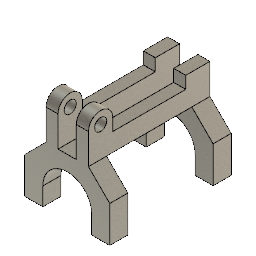
ch4Excercises v7 (Autodesk Fusion 360 design; units mm, degrees)
Autodesk Fusion 360 part; units mm, degrees
note: some values were not read from the file. Chosen so that the rebuilt part matches the saved one: which face or edge a step refers to.
sketch "Sketch1" plane through (0, 0, 0) normal (0, 0, 1) x (1, 0, 0) in component "ch4-1"
  line L0 (0, 0) -> (25.4, 0)
  line L1 (25.4, 0) -> (31.75, 6.35)
  line L2 (25.4, 0) -> (41.3581, 0) construction
  line L3 (31.75, 6.35) -> (31.75, 9.525)
  line L4 (31.75, 9.525) -> (19.05, 9.525)
  line L5 (19.05, 9.525) -> (19.05, 5.08)
  line L6 (0, 0) -> (-6.35, 6.35)
  line L7 (0, 0) -> (10.2611, 0) construction
  line L8 (-6.35, 6.35) -> (-6.35, 25.4)
  line L9 (-6.35, 25.4) -> (0, 31.75)
  line L10 (0, 31.75) -> (25.4, 31.75)
  line L11 (25.4, 31.75) -> (31.75, 25.4)
  line L12 (25.4, 31.75) -> (30.3579, 31.75) construction
  line L13 (31.75, 25.4) -> (31.75, 22.225)
  line L14 (31.75, 22.225) -> (19.05, 22.225)
  line L15 (19.05, 22.225) -> (19.05, 26.67)
  line L16 (19.05, 26.67) -> (4.445, 26.67)
  line L17 (4.445, 26.67) -> (1.27, 23.495)
  line L18 (1.27, 23.495) -> (1.27, 8.255)
  line L19 (1.27, 8.255) -> (4.445, 5.08)
  line L20 (4.445, 5.08) -> (19.05, 5.08)
  dimension "d17" = 25.4
  dimension "d18" = 45
  dimension "d20" = 6.35
  dimension "d21" = 9.525
  dimension "d22" = 12.7
  dimension "d23" = 5.08
  dimension "d24" = 135
  dimension "d26" = 6.35
  dimension "d27" = 6.35
  dimension "d28" = 31.75
  dimension "d29" = 31.75
  dimension "d30" = 45
  dimension "d32" = 6.35
  dimension "d33" = 12.7
  dimension "d34" = 5.08
  dimension "d35" = 7.62
  dimension "d36" = 3.175
  dimension "d37" = 135
  dimension "d38" = 3.175
  dimension "d39" = 135
  measures "d18" angle of L1 L2
  measures "d23" distance of L0.start
  measures "d24" angle of L6 L7
  measures "d26" distance of L0.start
  measures "d28" distance of L0.start
  measures "d29" distance of L0.start
  measures "d30" angle of L11 L12
  measures "d33" distance of L0.start
  measures "d34" distance of L10
  measures "d37" angle of L16 L17
  measures "d39" angle of L18 L19
extrude "Extrude1" add sketch "Sketch1" along normal blind 6.35 makes body 1 in component "ch4-1"
chamfer "Chamfer1" distance 0.127 angle 45 36 edges at (25.4, 22.225, 6.35) (31.75, 23.8125, 6.35) (28.575, 28.575, 6.35) (12.7, 31.75, 6.35) (11.7475, 26.67, 6.35) (2.8575, 25.0825, 6.35) (1.27, 15.875, 6.35) (2.8575, 6.6675, 6.35) (19.05, 7.3025, 6.35) (11.7475, 5.08, 6.35) (25.4, 9.525, 6.35) (31.75, 7.9375, 6.35) (28.575, 3.175, 6.35) (12.7, 0, 6.35) (-3.175, 3.175, 6.35) (-6.35, 15.875, 6.35) (-3.175, 28.575, 6.35) (12.7, 0, 0) (-3.175, 3.175, 0) (-6.35, 15.875, 0) (-3.175, 28.575, 0) (12.7, 31.75, 0) (2.8575, 25.0825, 0) (1.27, 15.875, 0) (2.8575, 6.6675, 0) (11.7475, 5.08, 0) (19.05, 7.3025, 0) (25.4, 9.525, 0) (31.75, 7.9375, 0) (28.575, 3.175, 0) (28.575, 28.575, 0) (31.75, 23.8125, 0) (25.4, 22.225, 0) (19.05, 24.4475, 0) (11.7475, 26.67, 0) (19.05, 24.4475, 6.35) on bodies 1 in component "ch4-1"
sketch "Sketch1 (2)" plane through (0, 0, 0) normal (0, 0, 1) x (1, 0, 0) in component "ch4-2"
  line L0 (0, 0) -> (-127, 0)
  line L1 (-127, 0) -> (-127, 136.525)
  line L2 (-127, 136.525) -> (0, 136.525)
  line L3 (0, 136.525) -> (0, 0)
  dimension "d43" = 127
  dimension "d44" = 136.525
extrude "Extrude1'" add sketch "Sketch1 (2)" along normal blind 34.925 separate body makes body 2 in component "ch4-2"
sketch "Sketch3" plane through (0, 0, 0) normal (0, -1, 0) x (1, 0, 0) in component "ch4-2"
  line L0 (-127, 0) -> (0, 0)
  line L1 (0, 0) -> (0, 34.925)
  line L2 (0, 34.925) -> (-127, 34.925)
  line L3 (-127, 34.925) -> (-127, 0)
  line L4 (-101.6, 0) -> (-25.4, 0)
  line L5 (-25.4, 0) -> (-25.4, 3.175)
  line L6 (-25.4, 3.175) -> (-101.6, 3.175)
  line L7 (-101.6, 3.175) -> (-101.6, 0)
  dimension "d47" = 76.2
  dimension "d48" = 3.175
  measures "d48" distance of L0.end
extrude "Extrude2" cut sketch "Sketch3" against normal through all contours L0 L4 L5 L6 L7 bodies 2 in component "ch4-2"
sketch "Sketch2" plane through (0, 0, 34.925) normal (0, 0, 1) x (-1, 0, 0) in component "ch4-2"
  line L0 (0, -136.525) -> (127, -136.525)
  line L1 (127, -136.525) -> (127, 0)
  line L2 (127, 0) -> (0, 0)
  line L3 (0, 0) -> (0, -136.525)
  line L4 (127, -136.525) -> (0, -136.525)
  line L5 (0, -136.525) -> (0, -104.775)
  line L6 (0, -104.775) -> (127, -104.775)
  line L7 (127, -104.775) -> (127, -136.525)
  dimension "d50" = 127
  dimension "d51" = 31.75
extrude "Extrude3" add sketch "Sketch2" along normal blind 101.6 contours L0 L1 L3 L4 L5 L6 L7 bodies 2 in component "ch4-2"
sketch "Sketch4" plane through (0, 0, 34.925) normal (0, 0, 1) x (-1, 0, 0) in component "ch4-2"
  line L0 (0, -104.775) -> (127, -104.775)
  line L1 (127, -104.775) -> (127, 0)
  line L2 (127, 0) -> (0, 0)
  line L3 (0, 0) -> (0, -104.775)
  line L4 (127, 0) -> (95.25, 0)
  line L5 (95.25, 0) -> (95.25, -28.575)
  line L6 (95.25, -28.575) -> (127, -28.575)
  line L7 (127, -28.575) -> (127, 0)
  dimension "d54" = 31.75
  dimension "d55" = 28.575
extrude "Extrude4" add sketch "Sketch4" along normal blind 9.525 contours L1 L2 L4 L5 L6 L7 bodies 2 in component "ch4-2"
ref_plane "WorkPlane1" through (-63.5, 68.2625, 68.2625) normal (1, 0, 0) x (0, 1, 0) in component "ch4-2"
mirror "Mirror1" about plane through (-63.5, 68.2625, 68.2625) normal (1, 0, 0) of "Extrude4" in component "ch4-2"
hole "Hole1" at (-63.5, 104.775, 85.725) direction (0, 1, 0) diameter 50.8 depth 31.75 tip angle 118 bodies 2 in component "ch4-2"
fillet "Fillet1" radius 12.7 3 edges at (0, 120.65, 136.525) (-127, 120.65, 136.525) (-63.5, 104.775, 34.925) on bodies 2 in component "ch4-2"
sketch "Sketch1 (3)" plane through (0, 0, 0) normal (0, 0, 1) x (1, 0, 0) in component "ch4-3"
  line L0 (0, 0) -> (88.9, 0)
  line L1 (88.9, 0) -> (88.9, 76.2)
  line L2 (88.9, 76.2) -> (0, 76.2)
  line L3 (0, 76.2) -> (0, 0)
  dimension "d65" = 76.2
  dimension "d66" = 88.9
extrude "Extrude1''" add sketch "Sketch1 (3)" along normal blind 44.45 separate body makes body 3 in component "ch4-3"
sketch "Sketch2 (2)" plane through (0, 0, 0) normal (0, -1, 0) x (1, 0, 0) in component "ch4-3"
  line L0 (0, 0) -> (88.9, 0)
  line L1 (88.9, 0) -> (88.9, 44.45)
  line L2 (88.9, 44.45) -> (0, 44.45)
  line L3 (0, 44.45) -> (0, 0)
  line L4 (0, 0) -> (19.05, 0)
  line L5 (19.05, 0) -> (19.05, 12.7)
  line L6 (19.05, 12.7) -> (0, 12.7)
  line L7 (0, 12.7) -> (0, 0)
  dimension "d69" = 12.7
  dimension "d70" = 19.05
  measures "d69" distance of L0.start
  measures "d70" distance of L0.start
extrude "Extrude2'" cut sketch "Sketch2 (2)" against normal through all contours L0 L3 L4 L5 L6 L7 bodies 3 in component "ch4-3"
sketch "Sketch3 (2)" plane through (0, 0, 0) normal (0, -1, 0) x (1, 0, 0) in component "ch4-3"
  line L0 (19.05, 12.7) -> (19.05, 0)
  line L1 (19.05, 0) -> (88.9, 0)
  line L2 (88.9, 0) -> (88.9, 44.45)
  line L3 (88.9, 44.45) -> (0, 44.45)
  line L4 (0, 44.45) -> (0, 12.7)
  line L5 (0, 12.7) -> (19.05, 12.7)
  line L6 (88.9, 0) -> (114.3, 31.75)
  line L7 (114.3, 31.75) -> (114.3, 44.45)
  line L8 (114.3, 44.45) -> (88.9, 44.45)
  dimension "d72" = 12.7
  dimension "d73" = 25.4
extrude "Extrude3'" add sketch "Sketch3 (2)" against normal up to surface (76.2 mm away) contours L2 L6 L7 L8 bodies 3 in component "ch4-3"
sketch "Sketch4 (2)" plane through (0, 0, 0) normal (0, -1, 0) x (1, 0, 0) in component "ch4-3"
  line L0 (19.05, 12.7) -> (19.05, 0)
  line L1 (19.05, 0) -> (88.9, 0)
  line L2 (88.9, 0) -> (114.3, 31.75)
  line L3 (114.3, 31.75) -> (114.3, 44.45)
  line L4 (114.3, 44.45) -> (0, 44.45)
  line L5 (0, 44.45) -> (0, 12.7)
  line L6 (0, 12.7) -> (19.05, 12.7)
  line L7 (0, 44.45) -> (0, 120.65)
  line L8 (-30.7418, 52.3875) -> (-12.2967, 123.825)
  line L9 (0, 120.65) -> (0, 133.35)
  line L10 (0, 44.45) -> (0, 12.7)
  arc A0 (0, 133.35) -> (-12.2967, 123.825) centre (0, 120.65) ccw
  arc A1 (-30.7418, 52.3875) -> (0, 12.7) centre (0, 44.45) ccw
  dimension "d76" = 76.2
  dimension "d77" = 25.4
  dimension "d78" = 63.5
  measures "d77" diameter of A0
  measures "d78" diameter of A1
extrude "Extrude4'" add sketch "Sketch4 (2)" against normal up to surface (76.2 mm away) contours L5 L7 L8 L9 L10 A0 A1 bodies 3 in component "ch4-3"
sketch "Sketch5" plane through (0, 0, 44.45) normal (0, 0, 1) x (-1, 0, 0) in component "ch4-3"
  line L0 (0, -76.2) -> (0, 0)
  line L1 (0, 0) -> (-114.3, 0)
  line L2 (-114.3, 0) -> (-114.3, -76.2)
  line L3 (-114.3, -76.2) -> (0, -76.2)
  circle A0 centre (-50.8, -38.1) radius 38.1
  dimension "d81" = 50.8
  dimension "d82" = 76.2
  measures "d82" diameter of A0
extrude "Extrude5" cut sketch "Sketch5" against normal blind 12.7 contours L1 L2 L3 A0 bodies 3 in component "ch4-3"
hole "Hole1'" at (50.8, 38.1, 44.45) direction (0, 0, -1) diameter 38.1 depth 44.45 tip angle 118 bodies 3 in component "ch4-3"
sketch "Sketch1 (4)" plane through (0, 0, 0) normal (0, 1, 0) x (1, 0, 0) in component "ch4-1 (1)"
  line L0 (0, 0) -> (0, -38.1)
  line L1 (0, -38.1) -> (22.225, -60.325)
  line L2 (22.225, -60.325) -> (22.225, -92.075)
  line L3 (22.225, -92.075) -> (34.925, -92.075)
  line L4 (34.925, -92.075) -> (34.925, -60.325)
  line L5 (34.925, -60.325) -> (53.975, -60.325)
  line L6 (53.975, -60.325) -> (53.975, -92.075)
  line L7 (53.975, -92.075) -> (66.675, -92.075)
  line L8 (66.675, -92.075) -> (66.675, -60.325)
  line L9 (88.9, 0) -> (88.9, -38.1)
  line L10 (88.9, -38.1) -> (66.675, -60.325)
  line L11 (88.9, 0) -> (69.85, 0)
  line L12 (0, 0) -> (19.05, 0)
  line L13 (19.05, 0) -> (19.05, -19.05)
  line L14 (19.05, -19.05) -> (69.85, -19.05)
  line L15 (69.85, 0) -> (69.85, -19.05)
  dimension "d88" = 38.1
  dimension "d89" = 31.75
  dimension "d90" = 12.7
  dimension "d91" = 19.05
  dimension "d92" = 12.7
  dimension "d93" = 38.1
  dimension "d94" = 45
  dimension "d95" = 45
  dimension "d96" = 31.75
  dimension "d97" = 19.05
  dimension "d98" = 19.05
  dimension "d99" = 19.05
  dimension "d100" = 50.8
  dimension "d101" = 19.05
  measures "d94" angle of L9 L10
  measures "d95" angle of L0 L1
  measures "d98" distance of L0.start
  measures "d101" distance of L0.start
extrude "Extrude1'''" add sketch "Sketch1 (4)" along normal blind 127 separate body makes body 4 in component "ch4-1 (1)"
sketch "Sketch2 (3)" plane through (88.9, 0, 0) normal (1, 0, 0) x (0, 1, 0) in component "ch4-1 (1)"
  line L0 (0, 38.1) -> (0, 0)
  line L1 (0, 0) -> (127, 0)
  line L2 (127, 0) -> (127, 38.1)
  line L3 (127, 38.1) -> (0, 38.1)
  line L4 (19.05, 60.325) -> (107.95, 60.325)
  line L5 (107.95, 60.325) -> (107.95, 0)
  line L6 (107.95, 0) -> (19.05, 0)
  line L7 (19.05, 0) -> (19.05, 60.325)
  line L8 (0, 60.325) -> (127, 60.325)
  dimension "d104" = 88.9
  measures "d104" distance of L0.end
extrude "Extrude2''" cut sketch "Sketch2 (3)" against normal through all contours L3 L4 L5 L7 L8 | L1 L3 L5 L6 L7 bodies 4 in component "ch4-1 (1)"
sketch "Sketch3 (3)" plane through (66.675, 0, 0) normal (1, 0, 0) x (0, 1, 0) in component "ch4-1 (1)"
  line L0 (0, 92.075) -> (0, 60.325)
  line L1 (0, 60.325) -> (19.05, 60.325)
  line L2 (19.05, 60.325) -> (107.95, 60.325)
  line L3 (107.95, 60.325) -> (127, 60.325)
  line L4 (127, 60.325) -> (127, 92.075)
  line L5 (127, 92.075) -> (0, 92.075)
  line L6 (25.4, 92.075) -> (101.6, 92.075)
  line L7 (101.6, 92.075) -> (101.6, 79.375)
  line L8 (101.6, 79.375) -> (25.4, 79.375)
  line L9 (25.4, 79.375) -> (25.4, 92.075)
  dimension "d106" = 12.7
  dimension "d107" = 76.2
extrude "Extrude3''" cut sketch "Sketch3 (3)" against normal through all contours L5 L6 L7 L8 L9 bodies 4 in component "ch4-1 (1)"
sketch "Sketch4 (3)" plane through (66.675, 0, 0) normal (1, 0, 0) x (0, 1, 0) in component "ch4-1 (1)"
  line L0 (101.6, 92.075) -> (101.6, 79.375)
  line L1 (101.6, 79.375) -> (25.4, 79.375)
  line L2 (25.4, 79.375) -> (25.4, 92.075)
  line L3 (25.4, 92.075) -> (0, 92.075)
  line L4 (0, 92.075) -> (0, 60.325)
  line L5 (0, 60.325) -> (19.05, 60.325)
  line L6 (19.05, 60.325) -> (107.95, 60.325)
  line L7 (107.95, 60.325) -> (127, 60.325)
  line L8 (127, 60.325) -> (127, 92.075)
  line L9 (127, 92.075) -> (101.6, 92.075)
  circle A0 centre (12.7, 92.075) radius 12.7
extrude "Extrude4''" add sketch "Sketch4 (3)" against normal up to surface (12.7 mm away) contours L3 A0 picked at (15.3394, 97.8803) bodies 4 in component "ch4-1 (1)"
sketch "Sketch6" plane through (22.225, 0, 0) normal (-1, 0, 0) x (0, -1, 0) in component "ch4-1 (1)"
  line L0 (-101.6, 79.375) -> (-101.6, 92.075)
  line L1 (-101.6, 92.075) -> (-127, 92.075)
  line L2 (-127, 92.075) -> (-127, 60.325)
  line L3 (-127, 60.325) -> (-107.95, 60.325)
  line L4 (-107.95, 60.325) -> (-19.05, 60.325)
  line L5 (-19.05, 60.325) -> (0, 60.325)
  line L6 (0, 60.325) -> (0, 92.075)
  line L7 (0, 92.075) -> (-25.4, 92.075)
  line L8 (-25.4, 92.075) -> (-25.4, 79.375)
  line L9 (-25.4, 79.375) -> (-101.6, 79.375)
  arc A0 (0, 92.075) -> (-25.4, 92.075) centre (-12.7, 92.075) ccw
extrude "Extrude5'" add sketch "Sketch6" against normal up to surface (12.7 mm away) contours L7 A0 bodies 4 in component "ch4-1 (1)"
hole "Hole1''" at (66.675, 12.7, 92.075) direction (-1, 0, 0) diameter 12.7 depth 44.45 tip angle 118 bodies 4 in component "ch4-1 (1)"
sketch "Sketch1 (5)" plane through (0, 0, 0) normal (0, 0, 1) x (1, 0, 0) in component "ch4-5"
  line L0 (0, 0) -> (127, 0)
  line L1 (127, 0) -> (127, 44.45)
  line L2 (127, 44.45) -> (0, 44.45)
  line L3 (0, 44.45) -> (0, 0)
  dimension "d116" = 127
  dimension "d117" = 44.45
extrude "Extrude1''''" add sketch "Sketch1 (5)" along normal blind 38.1 separate body makes body 5 in component "ch4-5"
sketch "Sketch2 (4)" plane through (0, 0, 0) normal (0, -1, 0) x (1, 0, 0) in component "ch4-5"
  line L0 (0, 0) -> (127, 0)
  line L1 (127, 0) -> (127, 38.1)
  line L2 (127, 38.1) -> (0, 38.1)
  line L3 (0, 38.1) -> (0, 0)
  line L4 (12.7, 0) -> (114.3, 0)
  line L5 (114.3, 0) -> (114.3, 6.35)
  line L6 (114.3, 6.35) -> (12.7, 6.35)
  line L7 (12.7, 6.35) -> (12.7, 0)
  dimension "d120" = 101.6
  dimension "d121" = 6.35
  measures "d120" distance of L0.start
extrude "Extrude2'''" cut sketch "Sketch2 (4)" against normal through all contours L0 L4 L5 L6 L7 bodies 5 in component "ch4-5"
sketch "Sketch3 (4)" plane through (0, 0, 38.1) normal (0, 0, 1) x (-1, 0, 0) in component "ch4-5"
  line L0 (0, -44.45) -> (0, 0)
  line L1 (0, 0) -> (-127, 0)
  line L2 (-127, 0) -> (-127, -44.45)
  line L3 (-127, -44.45) -> (0, -44.45)
  line L4 (-9.525, -44.45) -> (-117.475, -44.45)
  line L5 (-117.475, -44.45) -> (-117.475, 0)
  line L6 (-117.475, 0) -> (-9.525, 0)
  line L7 (-9.525, 0) -> (-9.525, -44.45)
  dimension "d123" = 107.95
  measures "d123" distance of L0.end
extrude "Extrude3'''" add sketch "Sketch3 (4)" along normal blind 38.1 contours L1 L3 L4 L5 L6 L7 bodies 5 in component "ch4-5"
sketch "Sketch4 (4)" plane through (0, 0, 0) normal (0, -1, 0) x (1, 0, 0) in component "ch4-5"
  line L0 (12.7, 0) -> (12.7, 6.35)
  line L1 (12.7, 6.35) -> (114.3, 6.35)
  line L2 (114.3, 6.35) -> (114.3, 0)
  line L3 (114.3, 0) -> (127, 0)
  line L4 (127, 0) -> (127, 38.1)
  line L5 (127, 38.1) -> (117.475, 38.1)
  line L6 (117.475, 38.1) -> (117.475, 76.2)
  line L7 (117.475, 76.2) -> (9.525, 76.2)
  line L8 (9.525, 76.2) -> (9.525, 38.1)
  line L9 (9.525, 38.1) -> (0, 38.1)
  line L10 (0, 38.1) -> (0, 0)
  line L11 (0, 0) -> (12.7, 0)
  circle A0 centre (63.5, 76.2) radius 53.975
extrude "Extrude4'''" add sketch "Sketch4 (4)" against normal up to surface (44.45 mm away) contours L7 A0 picked at (59.4965, 93.7406) bodies 5 in component "ch4-5"
hole "Hole1'''" at (63.5, 0, 76.2) direction (0, 1, 0) diameter 63.5 depth 44.45 tip angle 118 bodies 5 in component "ch4-5"
sketch "Sketch5 (2)" plane through (0, 0, 0) normal (0, -1, 0) x (1, 0, 0) in component "ch4-5"
  circle A0 centre (63.5, 76.2) radius 31.75
  line L0 (12.7, 0) -> (12.7, 6.35)
  line L1 (12.7, 6.35) -> (114.3, 6.35)
  line L2 (114.3, 6.35) -> (114.3, 0)
  line L3 (114.3, 0) -> (127, 0)
  line L4 (127, 0) -> (127, 38.1)
  line L5 (127, 38.1) -> (117.475, 38.1)
  line L6 (117.475, 38.1) -> (117.475, 76.2)
  arc A1 (117.475, 76.2) -> (9.525, 76.2) centre (63.5, 76.2) ccw
  line L7 (9.525, 76.2) -> (9.525, 38.1)
  line L8 (9.525, 38.1) -> (0, 38.1)
  line L9 (0, 38.1) -> (0, 0)
  line L10 (0, 0) -> (12.7, 0)
  line L11 (127, 38.1) -> (114.3, 38.1)
  line L12 (114.3, 38.1) -> (114.3, 94.439)
  line L13 (114.3, 94.439) -> (127, 94.439)
  line L14 (127, 94.439) -> (127, 38.1)
  dimension "d131" = 12.7
extrude "Extrude5''" cut sketch "Sketch5 (2)" against normal through all contours L6 A1 L11 L12 bodies 5 in component "ch4-5"
ref_plane "WorkPlane1" through (63.5, 22.225, 19.05) normal (1, 0, 0) x (0, 1, 0) in component "ch4-5"
mirror "Mirror1'" about plane through (63.5, 22.225, 19.05) normal (1, 0, 0) of "Extrude5''" in component "ch4-5"
sketch "Sketch1 (6)" plane through (0, 0, 0) normal (0, 0, 1) x (1, 0, 0) in component "ch4-6"
  circle A0 centre (0, 0) radius 19.05
  dimension "d134" = 38.1
  measures "d134" diameter of A0
extrude "Extrude1'''''" add sketch "Sketch1 (6)" along normal blind 25.4 separate body makes body 6 in component "ch4-6"
sketch "Sketch2 (5)" plane through (0, 0, 25.4) normal (0, 0, 1) x (-1, 0, 0) in component "ch4-6"
  circle A0 centre (0, 0) radius 19.05
  line L0 (0.1309, -19.0495) -> (-44.3191, -19.0495)
  line L1 (-44.3191, -19.0495) -> (-44.3191, -3.8095)
  line L2 (-44.3191, -3.8095) -> (0.1309, -3.8095)
  line L3 (0.1309, -3.8095) -> (0.1309, -19.0495)
  dimension "d137" = 44.45
  dimension "d138" = 15.24
extrude "Extrude2''''" add sketch "Sketch2 (5)" against normal blind 6.35 contours A0 L0 L1 L2 bodies 6 in component "ch4-6"
hole "Hole1''''" at (0, 0, 25.4) direction (0, 0, -1) diameter 19.05 depth 25.4 tip angle 118 bodies 6 in component "ch4-6"
hole "Hole2" at (34.1591, 11.4295, 25.4) direction (0, 0, -1) diameter 6.35 depth 6.35 tip angle 118 bodies 6 in component "ch4-6"
ref_plane "WorkPlane1" through (22.225, -19.0505, 22.225) normal (0, 1, 0) x (1, 0, 0) in component "ch4-6"
sketch "Sketch3 (5)" plane through (22.225, -19.0505, 22.225) normal (0, 1, 0) x (1, 0, 0) in component "ch4-6"
  line L0 (-12.7, -3.175) -> (-31.75, -3.175) construction
  line L1 (-41.275, 22.225) -> (-3.175, 22.225) construction
  line L2 (-22.225, -3.175) -> (-22.225, 22.225) construction
  circle A0 centre (-22.225, 9.525) radius 3.175
  dimension "d150" = 6.35
  measures "d150" diameter of A0
extrude "Extrude3''''" cut sketch "Sketch3 (5)" along normal up to surface end surface at (0.9484, -9.4777, 16.9333) on bodies 6 bodies 6 in component "ch4-6"
fillet "Fillet1'" radius 3.175 3 edges at (18.6652, 3.8095, 22.225) (44.3191, 3.8095, 22.225) (44.3191, 19.0495, 22.225) on bodies 6 in component "ch4-6"
hole "Hole2'" at (44.45, 0, 19.05) direction (0, 1, 0) diameter 50.8 depth 127 tip angle 118 bodies 4 in component "ch4-1 (1)"
component "ch4-1" placed x (1, 0, 0) y (0, 1, 0) z (0, 0, 1) at (0, 0, 0)
component "ch4-2" placed x (1, 0, 0) y (0, 1, 0) z (0, 0, 1) at (0, 0, 0)
component "ch4-3" placed x (1, 0, 0) y (0, 1, 0) z (0, 0, 1) at (0, 0, 0)
component "ch4-1 (1)" placed x (1, 0, 0) y (0, 1, 0) z (0, 0, 1) at (0, 0, 0)
component "ch4-5" placed x (1, 0, 0) y (0, 1, 0) z (0, 0, 1) at (0, 0, 0)
component "ch4-6" placed x (1, 0, 0) y (0, 1, 0) z (0, 0, 1) at (0, 0, 0)
equation "d45 = 1.75 in - 0.375 in"
equation "d52 = 5.375 in - 1.75 in + 0.375 in"
equation "d55 = 5.375 in - 3 in - 1.25 in"
equation "d104 = 5 in - 0.75 in - 0.75 in"
equation "d134 = ( 0.75 * 2 ) * 1 in"
